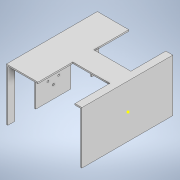
# Autodesk Inventor part: intakeCover
Saved by Autodesk Inventor 2020 (Build 240168000, 168)
## iProperties
Created: 2019-10-18
Part Number: intakeCover
Material: Generic
Document SubType Name: Modeling
Designer: tdmp4
Density: 1 g/cm^3
Appearance: Default
Author: tdmp4
Autodesk Inventor part; units mm, degrees
ref_plane "YZ Plane" through (0, 0, 0) normal (1, 0, 0) x (0, 1, 0)
ref_plane "XZ Plane" through (0, 0, 0) normal (0, 1, 0) x (-1, 0, 0)
ref_plane "XY Plane" through (0, 0, 0) normal (0, 0, 1) x (1, 0, 0)
sketch "Sketch1" plane through (0, 0, 0) normal (1, 0, 0) x (0, 1, 0)
  line L0 (-47.625, 82.55) -> (-47.625, -82.55)
  line L1 (-47.625, -82.55) -> (47.625, -82.55)
  line L2 (47.625, -82.55) -> (47.625, 82.55)
  line L3 (47.625, 82.55) -> (-47.625, 82.55)
  line L4 (-47.625, 82.55) -> (47.625, -82.55) construction
  line L5 (-47.625, -82.55) -> (47.625, 82.55) construction
  point P0 (0, 0)
  dimension "d0" = 165.1
  dimension "d1" = 95.25
  constraints: 12 end point, 2 midpoint, 2 parallel, 1 perpendicular, 1 vertical
  measures "d0" distance of L0.start L0.end
  measures "d1" distance of L1.end L0.end
extrude "Extrusion1" add sketch "Sketch1" along normal mid plane 138.43
sketch "Sketch3" plane through (-69.215, 47.625, 82.55) normal (0, 1, 0) x (1, 0, 0)
  line L0 (0, 0) -> (138.43, 0) projected
  line L1 (138.43, 0) -> (138.43, 82.55)
  line L2 (138.43, 165.1) -> (138.43, 0) projected
  line L3 (1.27, 63.5) -> (137.16, 63.5)
  line L4 (137.16, 63.5) -> (137.16, 101.6)
  line L5 (137.16, 101.6) -> (1.27, 101.6)
  line L6 (1.27, 101.6) -> (1.27, 63.5)
  line L7 (1.27, 63.5) -> (137.16, 101.6) construction
  line L8 (137.16, 63.5) -> (1.27, 101.6) construction
  line L9 (2.54, 0) -> (133.35, 0) projected
  line L10 (133.35, 0) -> (133.35, 63.5)
  line L11 (133.35, 0) -> (133.35, 165.1) projected
  line L12 (133.35, 63.5) -> (2.54, 63.5)
  line L13 (2.54, 63.5) -> (2.54, 0)
  line L14 (2.54, 0) -> (133.35, 0)
  line L15 (133.35, 0) -> (133.35, 63.5)
  line L16 (2.54, 165.1) -> (2.54, 0) projected
  line L17 (2.54, 165.1) -> (2.54, 101.6)
  line L18 (2.54, 101.6) -> (133.35, 101.6)
  line L19 (133.35, 101.6) -> (133.35, 165.1)
  line L20 (133.35, 165.1) -> (2.54, 165.1)
  line L21 (2.54, 165.1) -> (2.54, 101.6)
  point P0 (69.215, 82.55)
  point P1 (2.54, 101.6)
  point P2 (133.35, 101.6)
  dimension "d12" = 38.1
  dimension "d13" = 63.5
  constraints: 34 end point, 6 parallel, 3 horizontal, 3 midpoint, 3 perpendicular, 3 point on line
  measures "d12" distance of L4.end L3.end
  measures "d13" distance of L16.start L17.end
extrude "Extrusion3" cut sketch "Sketch3" against normal blind 12962.89 contours L13 L3 L10 L0 | L16 L20 L11 L5
sketch "Sketch4" plane through (69.215, 0, 0) normal (1, 0, 0) x (0, 0, -1)
  point P0 (0, 0)
sketch "Sketch5" plane through (-66.675, 47.625, 19.05) normal (0, 0, 1) x (1, 0, 0)
  line L0 (135.89, -95.25) -> (135.89, 0) projected
  line L1 (135.89, -95.25) -> (133.35, -95.25)
  line L2 (135.89, -95.25) -> (130.81, -95.25) projected
  line L3 (130.81, 0) -> (0, 0) projected
  line L4 (0, 0) -> (0, -2.54)
  line L5 (0, 0) -> (0, -95.25) projected
  line L6 (0, -2.54) -> (133.35, -2.54)
  line L7 (133.35, -2.54) -> (133.35, -95.25)
  line L8 (133.35, -95.25) -> (0, -95.25)
  line L9 (0, -95.25) -> (0, -2.54)
  point P0 (66.675, -47.625)
  dimension "d16" = 2.54
  dimension "d17" = 2.54
  constraints: 12 end point, 2 parallel, 1 horizontal, 1 midpoint, 1 perpendicular, 1 point on line
  measures "d16" distance of L0.start L1.end
  measures "d17" distance of L3.end L4.end
extrude "Extrusion4" cut sketch "Sketch5" along normal mid plane 203.2
sketch "Sketch7" plane through (-69.215, 47.625, 82.55) normal (0, 1, 0) x (1, 0, 0)
  line L0 (133.35, 63.5) -> (133.35, 0) projected
  line L1 (135.89, 0) -> (138.43, 0) projected
  line L2 (133.35, 63.5) -> (135.89, 63.5)
  line L3 (135.89, 63.5) -> (135.89, 0)
  line L4 (135.89, 0) -> (133.35, 0)
  line L5 (133.35, 0) -> (133.35, 63.5)
  line L6 (133.35, 101.6) -> (2.54, 101.6) projected
  line L7 (135.89, 0) -> (135.89, 165.1) projected
  line L8 (133.35, 101.6) -> (135.89, 101.6)
  line L9 (135.89, 101.6) -> (135.89, 165.1)
  line L10 (135.89, 165.1) -> (133.35, 165.1)
  line L11 (133.35, 165.1) -> (133.35, 101.6)
  point P0 (69.215, 82.55)
  constraints: 16 end point, 4 parallel, 2 horizontal, 2 perpendicular
extrude "Extrusion5" cut sketch "Sketch7" against normal blind 25.4
sketch "Sketch8" plane through (-69.215, 0, 0) normal (-1, 0, 0) x (0, 0, 1)
  line L0 (-19.05, 45.085) -> (19.05, 45.085) projected
  line L1 (-19.05, 45.085) -> (19.05, 45.085)
  line L2 (-19.05, 45.085) -> (-25.4, 45.085)
  line L3 (-25.4, 45.085) -> (-76.2, 45.085)
  line L4 (-25.4, 45.085) -> (-31.75, 45.085)
  line L5 (-82.55, -47.625) -> (82.55, -47.625) projected
  line L6 (-31.75, 45.085) -> (-31.75, -47.625)
  line L7 (-31.75, -47.625) -> (-69.85, -47.625)
  line L8 (-69.85, -47.625) -> (-69.85, 45.085)
  line L9 (-69.85, 45.085) -> (-31.75, 45.085)
  line L10 (19.05, 45.085) -> (31.75, 45.085)
  line L11 (31.75, 45.085) -> (31.75, -47.625)
  line L12 (31.75, -47.625) -> (69.85, -47.625)
  line L13 (69.85, -47.625) -> (69.85, 45.085)
  line L14 (69.85, 45.085) -> (31.75, 45.085)
  point P0 (0, 0)
  point P1 (-69.85, 45.085)
  dimension "d22" = 6.35
  dimension "d23" = 50.8
  dimension "d24" = 6.35
  dimension "d25" = 38.1
  dimension "d26" = 12.7
  dimension "d27" = 38.1
  constraints: 26 end point, 5 equal length, 5 point on line, 3 perpendicular, 1 horizontal, 1 vertical
  measures "d22" distance of L0.start L2.end
  measures "d23" distance of L2.end L3.end
  measures "d24" distance of L2.end L4.end
  measures "d25" distance of L6.end L7.end
  measures "d26" distance of L0.end L10.end
  measures "d27" distance of L12.end L11.end
extrude "Extrusion6" cut sketch "Sketch8" against normal blind 25.4 contours L14 L13 L5 L11 | L6 L5 L8 L3
sketch "Sketch9" plane through (-69.215, 47.625, 82.55) normal (0, 1, 0) x (1, 0, 0)
  line L0 (2.54, 101.6) -> (2.54, 165.1) projected
  line L1 (2.54, 165.1) -> (2.54, 158.75)
  line L2 (2.54, 158.75) -> (135.89, 158.75)
  line L3 (135.89, 158.75) -> (135.89, 165.1)
  line L4 (135.89, 165.1) -> (2.54, 165.1)
  line L5 (2.54, 0) -> (2.54, 63.5) projected
  line L6 (2.54, 0) -> (2.54, 6.35)
  line L7 (2.54, 6.35) -> (135.89, 6.35)
  line L8 (135.89, 6.35) -> (135.89, 0)
  line L9 (135.89, 0) -> (2.54, 0)
  point P0 (69.215, 82.55)
  dimension "d30" = 6.35
  dimension "d31" = 6.35
  constraints: 16 end point, 4 parallel, 2 perpendicular, 2 point on line
  measures "d30" distance of L0.end L1.end
  measures "d31" distance of L5.start L6.end
extrude "Extrusion7" add sketch "Sketch9" against normal blind 2.54
sketch "Sketch10" plane through (-69.215, 0, 0) normal (-1, 0, 0) x (0, 0, 1)
  line L0 (-69.85, 45.085) -> (-69.85, -47.625) projected
  line L1 (-69.85, -47.625) -> (-69.85, 41.275)
  line L2 (-69.85, 41.275) -> (69.85, 41.275)
  line L3 (69.85, -47.625) -> (69.85, 45.085) projected
  line L4 (-69.85, 45.085) -> (-31.75, 45.085) projected
  line L5 (-69.85, 41.275) -> (-69.85, 45.085)
  line L6 (-69.85, 45.085) -> (-31.75, 45.085)
  line L7 (-31.75, 45.085) -> (-31.75, 41.275)
  line L8 (-31.75, 41.275) -> (-69.85, 41.275)
  line L9 (31.75, 45.085) -> (31.75, -47.625) projected
  line L10 (69.85, 45.085) -> (31.75, 45.085) projected
  line L11 (31.75, 41.275) -> (69.85, 41.275)
  line L12 (69.85, 41.275) -> (69.85, 45.085)
  line L13 (69.85, 45.085) -> (31.75, 45.085)
  line L14 (31.75, 45.085) -> (31.75, 41.275)
  point P0 (0, 0)
  dimension "d34" = 88.9
  constraints: 20 end point, 4 parallel, 4 perpendicular, 4 point on line, 1 horizontal
  measures "d34" distance of L0.end L1.end
extrude "Extrusion8" add sketch "Sketch10" against normal blind 2.54
sketch "Sketch11" plane through (-69.215, 47.625, 82.55) normal (0, 1, 0) x (1, 0, 0)
  line L0 (0, 165.1) -> (0, 152.4) projected
  line L1 (135.89, 101.6) -> (2.54, 101.6) projected
  line L2 (0, 158.75) -> (12.7, 158.75)
  line L3 (12.7, 158.75) -> (12.7, 101.6)
  line L4 (12.7, 101.6) -> (0, 101.6)
  line L5 (0, 101.6) -> (0, 158.75)
  line L6 (2.54, 63.5) -> (135.89, 63.5) projected
  line L7 (0, 6.35) -> (12.7, 6.35)
  line L8 (12.7, 6.35) -> (12.7, 63.5)
  line L9 (12.7, 63.5) -> (0, 63.5)
  line L10 (0, 63.5) -> (0, 6.35)
  line L11 (138.6414, 6.35) -> (125.9414, 6.35)
  line L12 (125.9414, 6.35) -> (125.9414, 63.5)
  line L13 (125.9414, 63.5) -> (138.6414, 63.5)
  line L14 (138.6414, 63.5) -> (138.6414, 6.35)
  line L15 (125.9414, 101.6) -> (138.6414, 101.6)
  line L16 (138.6414, 101.6) -> (138.6414, 158.75)
  line L17 (138.6414, 158.75) -> (125.9414, 158.75)
  line L18 (125.9414, 158.75) -> (125.9414, 101.6)
  point P0 (69.215, 82.55)
  dimension "d37" = 12.7
  dimension "d38" = 12.7
  dimension "d39" = 12.7
  constraints: 32 end point, 8 parallel, 7 point on line, 4 horizontal, 4 perpendicular, 1 midpoint
  measures "d37" distance of L3.end L4.end
  measures "d38" distance of L9.end L8.end
  measures "d39" distance of L12.end L13.end
extrude "Extrusion9" add sketch "Sketch11" against normal blind 2.54
sketch "Sketch12" plane through (-69.215, 47.625, -82.55) normal (0, 1, 0) x (1, 0, 0)
  line L0 (138.43, 0) -> (138.43, -6.35) projected
  line L1 (138.43, -6.35) -> (125.73, -6.35)
  line L2 (125.9414, -6.35) -> (12.7, -6.35) projected
  line L3 (138.43, -158.75) -> (138.43, -165.1) projected
  line L4 (138.43, -6.35) -> (138.43, -165.1)
  line L5 (138.43, -165.1) -> (125.73, -165.1)
  line L6 (125.73, -165.1) -> (125.73, -6.35)
  line L7 (125.73, -6.35) -> (138.43, -6.35)
  point P0 (69.215, -82.55)
  dimension "d42" = 12.7
  dimension "d43" = 12.7
  constraints: 10 end point, 2 parallel, 1 collinear, 1 perpendicular, 1 point on line
  measures "d42" distance of L0.end L1.end
  measures "d43" distance of L3.end L5.end
extrude "Extrusion10" add sketch "Sketch12" against normal blind 2.54
sketch "Sketch13" plane through (-69.215, 47.625, -82.55) normal (0, 1, 0) x (1, 0, 0)
  line L0 (125.73, -63.5) -> (125.73, -6.35) projected
  line L1 (12.7, -6.35) -> (125.73, -6.35) projected
  line L2 (125.73, -6.35) -> (12.7, -6.35)
  line L3 (12.7, -6.35) -> (12.7, 0)
  line L4 (12.7, 0) -> (125.73, 0)
  line L5 (125.73, 0) -> (125.73, -6.35)
  line L6 (125.73, -158.75) -> (125.73, -101.6) projected
  line L7 (12.7, -101.6) -> (12.7, -158.75) projected
  line L8 (125.73, -158.75) -> (12.7, -158.75)
  line L9 (12.7, -158.75) -> (12.7, -165.1)
  line L10 (12.7, -165.1) -> (125.73, -165.1)
  line L11 (125.73, -165.1) -> (125.73, -158.75)
  point P0 (69.215, -82.55)
  constraints: 16 end point, 4 parallel, 3 perpendicular, 1 horizontal
extrude "Extrusion11" cut sketch "Sketch13" against normal blind 2.54
sketch "Sketch14" plane through (-69.215, 0, 0) normal (-1, 0, 0) x (0, 0, 1)
  circle A0 centre (0, -5.2326) radius 1.7859
  circle A1 centre (9.779, -15.0116) radius 1.7859
  circle A2 centre (-9.779, -15.0116) radius 1.7859
  circle A3 centre (0, -24.7906) radius 1.7859
  point P0 (0, 0)
  dimension "d49" = 3.5719
  dimension "d50" = 3.5719
  dimension "d51" = 3.5719
  dimension "d52" = 3.5719
  constraints: 4 centre point
  measures "d49" diameter of A0
  measures "d50" diameter of A1
  measures "d51" diameter of A2
  measures "d52" diameter of A3
extrude "Extrusion12" cut sketch "Sketch14" against normal blind 2.54
sketch "Sketch15" plane through (-69.215, 47.625, 82.55) normal (0, 1, 0) x (1, 0, 0)
  line L0 (138.43, 158.75) -> (138.6414, 158.75) projected
  line L1 (138.43, 158.75) -> (138.6414, 158.75)
  line L2 (138.6414, 158.75) -> (138.6414, -0.8057)
  line L3 (138.6414, -0.8057) -> (138.43, -0.8057)
  line L4 (138.43, -0.8057) -> (138.43, 158.75)
  point P0 (69.215, 82.55)
  constraints: 8 end point, 3 equal length, 1 perpendicular
extrude "Extrusion13" cut sketch "Sketch15" against normal blind 152.4
sketch "Sketch16" plane through (69.215, 47.625, 82.55) normal (0, 1, 0) x (1, 0, 0)
  line L0 (-125.73, 101.6) -> (-125.73, 165.1) projected
  line L1 (-125.73, 165.1) -> (-81.28, 165.1)
  line L2 (-81.28, 165.1) -> (-81.28, 0)
  line L3 (-81.28, 0) -> (-125.73, 0)
  line L4 (-125.73, 0) -> (-125.73, 165.1)
  point P0 (-69.215, 82.55)
  dimension "d57" = 44.45
  constraints: 8 end point, 2 parallel, 1 horizontal, 1 perpendicular
  measures "d57" distance of L0.end L1.end
extrude "Extrusion14" add sketch "Sketch16" against normal blind 2.54
sketch "Sketch17" plane through (69.215, -47.625, -82.55) normal (0, 0, -1) x (-1, 0, 0)
  line L0 (2.54, 0) -> (0, 0) projected
  line L1 (0, 0) -> (1.27, 0)
  line L2 (1.27, 0) -> (3.81, 0)
  line L3 (3.81, 0) -> (3.81, 95.25)
  line L4 (3.81, 95.25) -> (1.27, 95.25)
  line L5 (1.27, 95.25) -> (1.27, 0)
  point P0 (69.215, 47.625)
  dimension "d60" = 1.27
  dimension "d61" = 2.54
  constraints: 10 end point, 2 parallel, 1 midpoint, 1 perpendicular, 1 point on line
  measures "d60" distance of L0.end L1.end
  measures "d61" distance of L1.end L2.end
extrude "Extrusion15" add sketch "Sketch17" against normal blind 165.1
sketch "Sketch18" plane through (69.215, -47.625, -82.55) normal (0, 0, -1) x (-1, 0, 0)
  line L0 (0, 0) -> (3.81, 0) projected
  line L1 (0, 0) -> (1.27, 0)
  line L2 (1.27, 0) -> (1.27, 95.25)
  line L3 (1.27, 95.25) -> (0, 95.25)
  line L4 (0, 95.25) -> (0, 0)
  point P0 (69.215, 47.625)
  dimension "d64" = 1.27
  constraints: 8 end point, 2 parallel, 1 perpendicular, 1 point on line
  measures "d64" distance of L0.start L1.end
extrude "Extrusion16" cut sketch "Sketch18" against normal blind 165.1
sketch "Sketch19" plane through (56.515, 47.625, -82.55) normal (-1, 0, 0) x (0, 0, 1)
  line L0 (0, -2.54) -> (0, 0) projected
  line L1 (101.6, 0) -> (165.1, 0) projected
  line L2 (0, 0) -> (165.1, 0)
  line L3 (165.1, 0) -> (165.1, -2.5502)
  line L4 (165.1, -2.5502) -> (0, -2.5502)
  line L5 (0, -2.5502) -> (0, 0)
  point P0 (82.55, -47.625)
  constraints: 8 end point, 2 parallel, 1 collinear, 1 perpendicular
extrude "Extrusion17" add sketch "Sketch19" along normal blind 1.27
equation "\"d49\" = d51"
body "Solid1"
